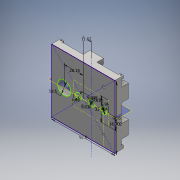
# Autodesk Inventor part: Lifting Platform With Balance
Saved by Autodesk Inventor 2016 (Build 200138000, 138)
## iProperties
Created: 2016-03-06
Part Number: Lifting Platform With Balance
Material: Generic
Document SubType Name: Modeling
Designer: Kenneth Daniel
Density: 1 g/cm^3
Appearance: Default
Author: Kenneth Daniel
Autodesk Inventor part; units mm, degrees
ref_plane "YZ Plane" through (0, 0, 0) normal (1, 0, 0) x (0, 1, 0)
ref_plane "XZ Plane" through (0, 0, 0) normal (0, 1, 0) x (-1, 0, 0)
ref_plane "XY Plane" through (0, 0, 0) normal (0, 0, 1) x (1, 0, 0)
sketch "Sketch1" plane through (0, 0, 0) normal (0, 1, 0) x (-1, 0, 0)
  line L0 (-46.4, 46.4) -> (-46.4, -46.4)
  line L1 (-46.4, -46.4) -> (46.4, -46.4)
  line L2 (46.4, -46.4) -> (46.4, 46.4)
  line L3 (46.4, 46.4) -> (-46.4, 46.4)
  line L4 (-46.4, 46.4) -> (46.4, -46.4) construction
  line L5 (-46.4, -46.4) -> (46.4, 46.4) construction
  circle A0 centre (28.15, 0) radius 9.75
  line L6 (-11.62, 56.3044) -> (-11.62, -68.4085) construction
  line L7 (13.88, 18.1678) -> (13.88, -16.702) construction
  line L8 (16.845, 0) -> (-37.12, 0) construction
  line L9 (-37.12, 0) -> (-37.12, -16.702) construction
  line L10 (-37.12, -16.702) -> (-37.12, 16.702) construction
  line L11 (-37.12, 16.702) -> (13.88, 16.702) construction
  line L12 (-37.12, -16.702) -> (13.88, -16.702) construction
  line L13 (13.88, 0) -> (6.92, 0) construction
  circle A1 centre (6.92, 0) radius 4.519 construction
  circle A2 centre (6.92, 0) radius 4.519
  circle A3 centre (-30.16, 0) radius 4.519
  circle A4 centre (-11.62, 0) radius 4.519
  point P0 (0, 0)
  dimension "d0" = 92.8
  dimension "d1" = 92.8
  dimension "d2" = 19.5
  dimension "d3" = 28.15
  dimension "d4" = 11.62
  dimension "d8" = 16.702
  dimension "d9" = 33.404
  dimension "d10" = 6.96
  dimension "d11" = 9.038
  dimension "d46" = 9.038
  dimension "d47" = 6.96
  dimension "d50" = 9.038
  constraints: 28 end point, 8 point on line, 5 centre point, 3 vertical, 2 coincident, 2 midpoint, 2 parallel, 2 perpendicular, 1 concentric
  measures "d0" distance of L0.start L0.end
  measures "d1" distance of L1.end L0.end
  measures "d2" diameter of A0
  measures "d3" distance of point (0, 0) A0.centre
  measures "d4" distance from line of L6 point (0, 0)
  measures "d8" distance of L8.end L9.end
  measures "d9" distance of L9.end L10.end
  measures "d10" distance of L13.start L13.end
  measures "d11" diameter of A1
  measures "d46" diameter of A3
  measures "d47" distance of L8.end A3.centre
  measures "d50" diameter of A4
extrude "Extrusion1" add sketch "Sketch1" along normal blind 10 contours L3 L2 L1 L0 | A3 | A4
sketch "Sketch2" plane through (0, 10, 0) normal (0, 1, 0) x (1, 0, 0)
  line L0 (-46.4, 46.4) -> (-46.4, -46.4) projected
  line L1 (46.4, -46.4) -> (46.4, 46.4) projected
  line L2 (-46.4, -46.4) -> (46.4, 46.4) construction
  line L3 (-46.4, 46.4) -> (46.4, -46.4) construction
  line L4 (-46.4, -44.4) -> (46.4, -44.4) construction
  line L5 (-46.4, 44.4) -> (46.4, 44.4) construction
  line L6 (46.4, 46.4) -> (-46.4, 46.4) construction
  line L7 (-43.9, 46.4) -> (-43.9, -46.4) construction
  line L8 (-46.4, -46.4) -> (46.4, -46.4) construction
  line L9 (43.9, -46.4) -> (43.9, 46.4) construction
  line L10 (-41.4, -42.4) -> (-46.4, -42.4)
  line L11 (-46.4, -42.4) -> (-46.4, -46.4)
  line L12 (-46.4, -46.4) -> (-41.4, -46.4)
  line L13 (-41.4, -46.4) -> (-41.4, -42.4)
  line L14 (-41.4, -42.4) -> (-46.4, -46.4) construction
  line L15 (-46.4, -42.4) -> (-41.4, -46.4) construction
  line L16 (-41.4, 42.4) -> (-46.4, 42.4)
  line L17 (-46.4, 42.4) -> (-46.4, 46.4)
  line L18 (-46.4, 46.4) -> (-41.4, 46.4)
  line L19 (-41.4, 46.4) -> (-41.4, 42.4)
  line L20 (-41.4, 42.4) -> (-46.4, 46.4) construction
  line L21 (-46.4, 42.4) -> (-41.4, 46.4) construction
  line L22 (41.4, 42.4) -> (46.4, 42.4)
  line L23 (46.4, 42.4) -> (46.4, 46.4)
  line L24 (46.4, 46.4) -> (41.4, 46.4)
  line L25 (41.4, 46.4) -> (41.4, 42.4)
  line L26 (41.4, 42.4) -> (46.4, 46.4) construction
  line L27 (46.4, 42.4) -> (41.4, 46.4) construction
  line L28 (41.4, -42.4) -> (46.4, -42.4)
  line L29 (46.4, -42.4) -> (46.4, -46.4)
  line L30 (46.4, -46.4) -> (41.4, -46.4)
  line L31 (41.4, -46.4) -> (41.4, -42.4)
  line L32 (41.4, -42.4) -> (46.4, -46.4) construction
  line L33 (46.4, -42.4) -> (41.4, -46.4) construction
  point P0 (0, 0)
  point P1 (-43.9, -44.4)
  point P2 (-43.9, 44.4)
  point P3 (43.9, 44.4)
  point P4 (43.9, -44.4)
  dimension "d14" = 2.5
  dimension "d15" = 2.5
  dimension "d16" = 2
  dimension "d17" = 2
  constraints: 60 end point, 16 point on line, 12 parallel, 8 midpoint, 8 perpendicular
  measures "d14" distance between parallel lines of L7 L0
  measures "d15" distance between parallel lines of L1 L9
  measures "d16" distance between parallel lines of L8 L4
  measures "d17" distance between parallel lines of L6 L5
extrude "Extrusion2" add sketch "Sketch2" along normal blind 3
sketch "Sketch3" plane through (-46.4, 0, 46.4) normal (0, 0, 1) x (1, 0, 0)
  line L0 (0, 10) -> (5, 10) construction
  line L1 (0, 10) -> (92.9772, 10) construction
  line L2 (0, 10) -> (0, 13) construction
  line L3 (5, 10) -> (0, 13) construction
  line L4 (0, 13) -> (5, 13) construction
  line L5 (5, 13) -> (0, 10) construction
  line L6 (92.8, 0) -> (92.8, 13) construction
  line L7 (87.8, 13) -> (92.8, 13) construction
  line L8 (92.8, 10) -> (87.8, 13) construction
  line L9 (87.8, 13) -> (87.8, 10) construction
  line L10 (87.8, 10) -> (92.8, 13) construction
  circle A0 centre (90.3, 11.5) radius 1 construction
  circle A1 centre (90.3, 11.5) radius 1
  circle A2 centre (2.5, 11.5) radius 1
  point P0 (46.4, 0)
  dimension "d20" = 2
  dimension "d21" = 2
  constraints: 14 end point, 3 centre point, 3 point on line, 2 midpoint, 2 perpendicular, 1 coincident, 1 concentric, 1 horizontal
  measures "d20" diameter of A0
  measures "d21" diameter of A2
sketch "Sketch4" plane through (0, 10, 0) normal (0, 1, 0) x (1, 0, 0)
  line L0 (0, -35.0564) -> (0, -55.3914) construction
  line L1 (-41.4, -46.4) -> (41.4, -46.4) projected
  line L2 (0, -46.4) -> (-10, -46.4)
  line L3 (-10, -46.4) -> (-10, -38.9)
  line L4 (-10, -38.9) -> (10, -38.9)
  line L5 (10, -38.9) -> (10, -46.4)
  line L6 (0, -46.4) -> (10, -46.4)
  line L7 (-23.157, 0) -> (-56.7416, 0) construction
  line L8 (-56.7416, 0) -> (-56.7416, -46.4) construction
  line L9 (-56.7416, -46.4) -> (-46.4, -46.4) construction
  line L10 (-46.4, -46.4) -> (-56.7416, -23.2) construction
  line L11 (-31.4038, -23.2) -> (-56.7416, -23.2) construction
  line L12 (-46.4, 42.4) -> (-46.4, -42.4) projected
  line L13 (-46.4, -23.2) -> (-46.4, -33.2)
  line L14 (-46.4, -33.2) -> (-38.9, -33.2)
  line L15 (-38.9, -33.2) -> (-38.9, -13.2)
  line L16 (-38.9, -13.2) -> (-46.4, -13.2)
  line L17 (-46.4, -13.2) -> (-46.4, -23.2)
  line L18 (-50.628, 0) -> (47.2568, 0) construction
  line L19 (0, -71.9527) -> (0, 59.9713) construction
  line L20 (46.4, -23.2) -> (46.4, -33.2)
  line L21 (46.4, -33.2) -> (38.9, -33.2)
  line L22 (38.9, -33.2) -> (38.9, -13.2)
  line L23 (38.9, -13.2) -> (46.4, -13.2)
  line L24 (46.4, -13.2) -> (46.4, -23.2)
  line L25 (0, 46.4) -> (-10, 46.4)
  line L26 (-10, 46.4) -> (-10, 38.9)
  line L27 (-10, 38.9) -> (10, 38.9)
  line L28 (10, 38.9) -> (10, 46.4)
  line L29 (0, 46.4) -> (10, 46.4)
  line L30 (-46.4, 23.2) -> (-46.4, 33.2)
  line L31 (-46.4, 33.2) -> (-38.9, 33.2)
  line L32 (-38.9, 33.2) -> (-38.9, 13.2)
  line L33 (-38.9, 13.2) -> (-46.4, 13.2)
  line L34 (-46.4, 13.2) -> (-46.4, 23.2)
  line L35 (46.4, 33.2) -> (38.9, 33.2)
  line L36 (38.9, 33.2) -> (38.9, 13.2)
  line L37 (38.9, 13.2) -> (46.4, 13.2)
  line L38 (46.4, 13.2) -> (46.4, 23.2)
  line L39 (46.4, 23.2) -> (46.4, 33.2)
  line L40 (9.3, -39.6) -> (-9.3, -39.6) construction
  line L41 (-9.3, -39.6) -> (-9.3, -45.7) construction
  line L42 (-9.3, -45.7) -> (0, -45.7) construction
  line L43 (0, -45.7) -> (9.3, -45.7) construction
  line L44 (9.3, -45.7) -> (9.3, -39.6) construction
  line L45 (-9.3, -39.6) -> (-9.3, -45.7)
  line L46 (-9.3, -45.7) -> (0, -45.7)
  line L47 (0, -45.7) -> (9.3, -45.7)
  line L48 (9.3, -45.7) -> (9.3, -39.6)
  line L49 (9.3, -39.6) -> (-9.3, -39.6)
  line L50 (-39.6, -13.9) -> (-39.6, -32.5)
  line L51 (-39.6, -32.5) -> (-45.7, -32.5)
  line L52 (-45.7, -32.5) -> (-45.7, -23.2)
  line L53 (-45.7, -23.2) -> (-45.7, -13.9)
  line L54 (-45.7, -13.9) -> (-39.6, -13.9)
  line L55 (-45.7, 13.9) -> (-39.6, 13.9)
  line L56 (-39.6, 13.9) -> (-39.6, 32.5)
  line L57 (-39.6, 32.5) -> (-45.7, 32.5)
  line L58 (-45.7, 32.5) -> (-45.7, 23.2)
  line L59 (-45.7, 23.2) -> (-45.7, 13.9)
  line L60 (9.3, 39.6) -> (-9.3, 39.6)
  line L61 (-9.3, 39.6) -> (-9.3, 45.7)
  line L62 (-9.3, 45.7) -> (0, 45.7)
  line L63 (0, 45.7) -> (9.3, 45.7)
  line L64 (9.3, 45.7) -> (9.3, 39.6)
  line L65 (39.6, 13.9) -> (39.6, 32.5)
  line L66 (39.6, 32.5) -> (45.7, 32.5)
  line L67 (45.7, 32.5) -> (45.7, 23.2)
  line L68 (45.7, 23.2) -> (45.7, 13.9)
  line L69 (45.7, 13.9) -> (39.6, 13.9)
  line L70 (39.6, -13.9) -> (39.6, -32.5)
  line L71 (39.6, -32.5) -> (45.7, -32.5)
  line L72 (45.7, -32.5) -> (45.7, -23.2)
  line L73 (45.7, -23.2) -> (45.7, -13.9)
  line L74 (45.7, -13.9) -> (39.6, -13.9)
  point P0 (0, 0)
  dimension "d22" = 10
  dimension "d23" = 7.5
  dimension "d24" = 20
  dimension "d25" = 10
  dimension "d26" = 7.5
  dimension "d27" = 20
  dimension "d28" = 0.7
  dimension "d29" = 0.7
  dimension "d30" = 0.7
  dimension "d31" = 0.7
  dimension "d32" = 0.7
  dimension "d33" = 0.7
  dimension "d34" = 0.7
  constraints: 146 end point, 20 symmetric about line, 15 perpendicular, 7 point on line, 3 vertical, 2 collinear, 2 horizontal, 2 midpoint, 28 other
  measures "d22" distance of L2.start L2.end
  measures "d23" distance of L2.end L3.end
  measures "d24" distance of L3.end L4.end
  measures "d25" distance of L13.start L13.end
  measures "d26" distance of L13.end L14.end
  measures "d27" distance of L14.end L15.end
  measures "d28" distance between parallel lines of L4 L40
  measures "d29" distance between parallel lines of L3 L45
  measures "d30" distance between parallel lines of L15 L50
  measures "d31" distance between parallel lines of L33 L55
  measures "d32" distance between parallel lines of L27 L60
  measures "d33" distance between parallel lines of L36 L65
  measures "d34" distance between parallel lines of L22 L70
extrude "Extrusion3" add sketch "Sketch4" along normal blind 10
extrude "Extrusion5" cut sketch "Sketch3" against normal blind 4
ref_plane "Work Plane1" through (46.4, 0, 0) normal (0, 0, -1) x (-1, 0, 0)
mirror "Mirror1" about plane through (46.4, 0, 0) normal (0, 0, -1) of "Extrusion5"
sketch "Sketch6" plane through (0, 10, 0) normal (0, 1, 0) x (1, 0, 0)
  circle A0 centre (-28.15, 0) radius 9.75 projected
  circle A1 centre (-6.92, 0) radius 4.519 projected
  line L0 (10, 46.4) -> (10, 38.9) projected
  line L1 (10, 38.9) -> (-10, 38.9) projected
  line L2 (-10, 38.9) -> (-10, 46.4) projected
  line L3 (-10, 46.4) -> (-41.4, 46.4) projected
  line L4 (-41.4, 46.4) -> (-41.4, 42.4) projected
  line L5 (-41.4, 42.4) -> (-46.4, 42.4) projected
  line L6 (-46.4, 42.4) -> (-46.4, 33.2) projected
  line L7 (-46.4, 33.2) -> (-38.9, 33.2) projected
  line L8 (-38.9, 33.2) -> (-38.9, 13.2) projected
  line L9 (-38.9, 13.2) -> (-46.4, 13.2) projected
  line L10 (-46.4, 13.2) -> (-46.4, -13.2) projected
  line L11 (-46.4, -13.2) -> (-38.9, -13.2) projected
  line L12 (-38.9, -13.2) -> (-38.9, -33.2) projected
  line L13 (-38.9, -33.2) -> (-46.4, -33.2) projected
  line L14 (-46.4, -33.2) -> (-46.4, -42.4) projected
  line L15 (-46.4, -42.4) -> (-41.4, -42.4) projected
  line L16 (-41.4, -42.4) -> (-41.4, -46.4) projected
  line L17 (-41.4, -46.4) -> (-10, -46.4) projected
  line L18 (-10, -46.4) -> (-10, -38.9) projected
  line L19 (-10, -38.9) -> (10, -38.9) projected
  line L20 (10, -38.9) -> (10, -46.4) projected
  line L21 (10, -46.4) -> (41.4, -46.4) projected
  line L22 (41.4, -46.4) -> (41.4, -42.4) projected
  line L23 (41.4, -42.4) -> (46.4, -42.4) projected
  line L24 (46.4, -42.4) -> (46.4, -33.2) projected
  line L25 (46.4, -33.2) -> (38.9, -33.2) projected
  line L26 (38.9, -33.2) -> (38.9, -13.2) projected
  line L27 (38.9, -13.2) -> (46.4, -13.2) projected
  line L28 (46.4, -13.2) -> (46.4, 13.2) projected
  line L29 (46.4, 13.2) -> (38.9, 13.2) projected
  line L30 (38.9, 13.2) -> (38.9, 33.2) projected
  line L31 (38.9, 33.2) -> (46.4, 33.2) projected
  line L32 (46.4, 33.2) -> (46.4, 42.4) projected
  line L33 (46.4, 42.4) -> (41.4, 42.4) projected
  line L34 (41.4, 42.4) -> (41.4, 46.4) projected
  line L35 (41.4, 46.4) -> (10, 46.4) projected
  point P0 (0, 0)
extrude "Extrusion7" add sketch "Sketch6" against normal blind 10 contours A1
extrude "Extrusion9" cut sketch "Sketch1" along normal blind 10 contours A4
sketch "Sketch7" plane through (0, 0, 0) normal (0, -1, 0) x (1, 0, 0)
  line L0 (30.16, 0) -> (30.16, -46.4) construction
  line L1 (41.4, -46.4) -> (10, -46.4) projected
  constraints: 2 end point, 1 point on line, 1 vertical
sketch "Sketch8" plane through (0, 0, 0) normal (0, -1, 0) x (1, 0, 0)
  circle A0 centre (11.62, 0) radius 4.519 projected
  circle A1 centre (-28.15, 0) radius 9.75 projected
  line L0 (46.4, 46.4) -> (46.4, -46.4) projected
  line L1 (-46.4, 46.4) -> (46.4, 46.4) projected
  line L2 (-46.4, -46.4) -> (-46.4, 46.4) projected
  line L3 (46.4, -46.4) -> (-46.4, -46.4) projected
  circle A2 centre (30.16, 0) radius 4.519 projected
  circle A3 centre (11.62, 0) radius 4.519 projected
  circle A4 centre (-28.15, 0) radius 9.75 projected
  line L4 (46.4, 46.4) -> (46.4, -46.4) projected
  line L5 (-46.4, 46.4) -> (46.4, 46.4) projected
  line L6 (-46.4, -46.4) -> (-46.4, 46.4) projected
  line L7 (46.4, -46.4) -> (-46.4, -46.4) projected
  line L8 (30.16, 0) -> (30.16, 46.8649) construction
  circle A5 centre (30.16, 30.1599) radius 1.6
  line L9 (55.9453, 0) -> (-55.3311, 0) construction
  line L10 (30.16, 0) -> (30.16, -46.8649) construction
  circle A6 centre (30.16, -30.1599) radius 1.6
  point P0 (0, 0)
  dimension "d53" = 3.2
  dimension "d54" = 30.1599
  dimension "d55" = 30.1599
  constraints: 6 end point, 2 centre point, 2 point on line, 2 symmetric about line, 1 coincident, 1 horizontal, 1 perpendicular, 1 other
  measures "d53" diameter of A5
  measures "d54" vertical distance of A0.centre A6.centre
  measures "d55" vertical distance of A0.centre A5.centre
extrude "Extrusion10" cut sketch "Sketch8" against normal up to surface (10 mm away) contours A5 | A6
body "Solid1"
